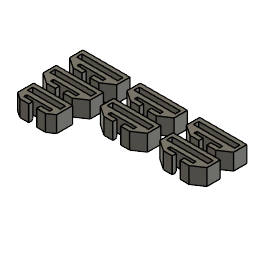
syringe pump (Autodesk Fusion 360 archive; units mm, degrees)
design "stringe pump 2"
Autodesk Fusion 360 part; units mm, degrees
sketch "Sketch1" plane through (0, 0, 0) normal (0, 1, 0) x (1, 0, 0)
  line L0 (0, 0) -> (19, 0)
  line L1 (19, -2.5) -> (0, -2.5)
  line L2 (0, 0) -> (19, 0)
  line L3 (-2, -4.5) -> (-2, 2)
  line L4 (-2, 2) -> (21, 2)
  line L5 (21, 2) -> (21, -4.5)
  line L6 (21, -4.5) -> (15.75, -8)
  line L7 (-2, -4.5) -> (3.25, -8)
  line L8 (15.75, -6) -> (15.75, -4.65)
  line L9 (3.25, -4.65) -> (3.25, -6)
  line L10 (3.25, -6) -> (7.5, -6)
  line L11 (15.75, -6) -> (11.5, -6)
  line L12 (3.25, -8) -> (7.5, -8)
  line L13 (11.5, -8) -> (15.75, -8)
  line L14 (3.25, -8) -> (7.5, -8)
  line L15 (11.5, -8) -> (15.75, -8)
  line L16 (15.75, -6) -> (11.5, -6)
  line L17 (7.5, -6) -> (3.25, -6)
  line L18 (3.25, -6) -> (7.5, -6)
  line L19 (11.5, -6) -> (15.75, -6)
  line L20 (7.5, -8) -> (11.5, -8)
  line L21 (15.75, -6) -> (15.75, -4.65)
  line L22 (15.75, -4.65) -> (3.25, -4.65)
  line L23 (3.25, -4.65) -> (3.25, -6)
  line L24 (0, 0) -> (-0.5, 0)
  line L25 (-0.5, 0) -> (-0.5, -2.5)
  line L26 (-0.5, -2.5) -> (-0.2, -2.5)
  line L27 (19, 0) -> (19.5, 0)
  line L28 (19.5, 0) -> (19.5, -2.5)
  line L29 (19.5, -2.5) -> (19, -2.5)
  line L30 (7.5, -6) -> (7.6, -6)
  line L31 (7.6, -6) -> (7.6, -8)
  line L32 (7.6, -8) -> (7.5, -8)
  line L33 (11.5, -6) -> (11.4, -6)
  line L34 (11.4, -6) -> (11.4, -8)
  line L35 (11.4, -8) -> (11.5, -8)
  line L36 (3.25, -6) -> (7.6, -6)
  line L37 (11.4, -6) -> (15.75, -6)
  line L38 (0, -2.5) -> (-0.2, -2.5)
  dimension "d28" = 1.35
  dimension "d29" = 0.5
  dimension "d30" = 0.5
  dimension "d31" = 0.1
  dimension "d32" = 0.1
  constraint horizontal L0
  constraint coincident L0.start L2.start
  constraint horizontal L2
  constraint vertical L3
  constraint horizontal L4
  constraint vertical L5
  constraint horizontal L12
  constraint horizontal L16
  constraint horizontal L18
  constraint vertical L8
  constraint vertical L9
  constraint collinear L16 L17
  constraint collinear L18 L19
  constraint horizontal L36
  constraint vertical L21
  constraint horizontal L22
  constraint vertical L23
  constraint horizontal L24
  constraint vertical L25
  constraint horizontal L26
  constraint horizontal L27
  constraint vertical L28
  constraint horizontal L29
  constraint horizontal L30
  constraint vertical L31
  constraint horizontal L32
  constraint horizontal L33
  constraint vertical L34
  constraint horizontal L35
  constraint collinear L36 L37
  constraint parallel L26 L38
  measures "d28" distance of L9.end L9.start
  measures "d29" distance of L0.start L24.end
  measures "d30" distance of L0.end L27.end
  measures "d31" distance of L10.end L30.end
  measures "d32" distance of L11.end L33.end
extrude "Extrude1" add sketch "Sketch1" along normal blind 8 contours L3 L4 L5 L6 L7 L8 L9 L10 L11 L12 L13 L14 L15 L16 L17 L18 L19 L20 L21 L22 L23 L30 L31 L32 L33 L34 L35 L36 L37 makes body 1
fillet "Fillet1" radius 2.5 1 edges at (9.5, 0, 0) on bodies 1
fillet "Fillet3" radius 1 2 edges at (9.5, 0, 2.5) (9.5, 0, 4.65) on bodies 1
fillet "Fillet2" radius 1 4 edges at (13.575, 0, 6) (5.425, 0, 6) (15.75, 0, 4.825) (3.25, 0, 4.825) on bodies 1
move_body "Move2" bodies 1 to x (1, 0, 0) y (0, 1, 0) z (0, 0, 1) at (0, 0, -17)
move_body "Move3" bodies 1 to x (1, 0, 0) y (0, 1, 0) z (0, 0, 1) at (-10, 0, 0)
copy_body "CopyPasteBodies1" bodies 1 makes body 2
move_body "Move4" bodies 2 to x (1, 0, 0) y (0, 1, 0) z (0, 0, 1) at (28, 0, 0)
copy_body "CopyPasteBodies2" bodies 2 makes body 3
move_body "Move5" bodies 3 to x (1, 0, 0) y (0, 1, 0) z (0, 0, 1) at (29, 0, 0)
copy_body "CopyPasteBodies3" bodies 1 2 3 makes body 4 makes body 5 makes body 6
move_body "Move6" bodies 4 5 6 to x (1, 0, 0) y (0, 1, 0) z (0, 0, 1) at (0, 0, 13)
copy_body "CopyPasteBodies4" bodies 1 makes body 7
move_body "Move7" bodies 7 to x (1, 0, 0) y (0, 1, 0) z (0, 0, 1) at (0, 0, 26)
sketch "Sketch2" plane through (0, 8, 0) normal (0, 1, 0) x (-1, 0, 0)
  line L0 (10.5, 9) -> (-9.5, 9)
  line L1 (-9.5, 9) -> (-9.5, 11.5)
  line L2 (-9.5, 11.5) -> (10.5, 11.5)
  line L3 (10.5, 11.5) -> (10.5, 9)
  line L4 (-1.4, 17) -> (-1.5, 17)
  line L5 (-1.5, 17) -> (-5.75, 17)
  line L6 (-5.75, 17) -> (-11, 13.5)
  line L7 (-11, 13.5) -> (-11, 7)
  line L8 (-11, 7) -> (12, 7)
  line L9 (12, 7) -> (12, 13.5)
  line L10 (12, 13.5) -> (6.75, 17)
  line L11 (6.75, 17) -> (2.5, 17)
  line L12 (2.5, 17) -> (2.4, 17)
  line L13 (2.4, 17) -> (2.4, 15)
  line L14 (2.4, 15) -> (6.75, 15)
  line L15 (6.75, 15) -> (6.75, 13.65)
  line L16 (6.75, 13.65) -> (-5.75, 13.65)
  line L17 (-5.75, 13.65) -> (-5.75, 15)
  line L18 (-5.75, 15) -> (-1.4, 15)
  line L19 (-1.4, 15) -> (-1.4, 17)
  line L20 (10.5, 7) -> (-9.5, 7)
  line L21 (-9.5, 7) -> (-9.5, 14.5)
  line L22 (-9.5, 14.5) -> (10.5, 14.5)
  line L23 (10.5, 14.5) -> (10.5, 7)
  line L24 (10.5, 7) -> (10, 7)
  line L25 (10, 7) -> (10, 14.5)
  line L26 (10, 14.5) -> (10.5, 14.5)
  line L27 (10.5, 14.5) -> (10.5, 7)
  line L28 (-9.5, 7) -> (-9, 7)
  line L29 (-9, 7) -> (-9, 14.5)
  line L30 (-9, 14.5) -> (-9.5, 14.5)
  line L31 (-9.5, 14.5) -> (-9.5, 7)
  line L32 (-9, 7) -> (-7.5, 7)
  line L33 (-7.5, 7) -> (-7.5, 12.5)
  line L34 (-7.5, 12.5) -> (-9, 12.5)
  line L35 (-9, 12.5) -> (-9, 7)
  line L36 (10, 7) -> (8.5, 7)
  line L37 (8.5, 7) -> (8.5, 12.5)
  line L38 (8.5, 12.5) -> (10, 12.5)
  line L39 (10, 12.5) -> (10, 7)
  line L40 (-9.5, 14.5) -> (-9, 14.5)
  line L41 (-9, 14.5) -> (-9, 15.5)
  line L42 (-9, 15.5) -> (-9.5, 15.5)
  line L43 (-9.5, 15.5) -> (-9.5, 14.5)
  line L44 (10.5, 14.5) -> (10, 14.5)
  line L45 (10, 14.5) -> (10, 15.5)
  line L46 (10, 15.5) -> (10.5, 15.5)
  line L47 (10.5, 15.5) -> (10.5, 14.5)
  dimension "d35" = 0.5
  dimension "d36" = 0.5
  dimension "d39" = 1.5
  dimension "d40" = 1.5
  dimension "d41" = 1
  constraint horizontal L20
  constraint vertical L21
  constraint horizontal L22
  constraint vertical L23
  constraint coincident L6 L21.end
  constraint coincident L8 L20.start
  constraint horizontal L24
  constraint vertical L25
  constraint horizontal L26
  constraint vertical L27
  constraint horizontal L28
  constraint vertical L29
  constraint horizontal L30
  constraint vertical L31
  constraint horizontal L32
  constraint vertical L33
  constraint horizontal L34
  constraint vertical L35
  constraint horizontal L36
  constraint vertical L37
  constraint horizontal L38
  constraint vertical L39
  constraint horizontal L40
  constraint vertical L41
  constraint horizontal L42
  constraint vertical L43
  constraint horizontal L44
  constraint vertical L45
  constraint horizontal L46
  constraint vertical L47
  measures "d35" distance of L20.start L24.end
  measures "d36" distance of L20.end L28.end
  measures "d39" distance of L28.end L32.end
  measures "d40" distance of L24.end L36.end
  measures "d41" distance of L22.end L46.end
extrude "Extrude3" cut sketch "Sketch2" against normal blind 8 contours L0 L8 L20 L23 L24 L25 L27 L39 | L0 L2 L3 L23 L25 L27 L39 | L3 L8 L9 L10 L23 L27 | L2 L22 L23 L25 L26 L27 L39 L44 | L10 L22 L26 L44 L45 | L10 L45 L46 L47 | L0 L8 L20 L21 L28 L29 L31 L35 | L0 L1 L2 L21 L29 L31 L35 | L1 L6 L7 L8 L21 L31 | L2 L21 L22 L29 L30 L31 L35 L40 | L6 L22 L30 L40 L41 | L6 L41 L42 L43 bodies 7 makes body 8 at (-3.6667, 2.6667, 7)
extrude "Extrude4" add sketch "Sketch2" against normal blind 8 contours L0 L8 L20 L25 L36 L37 L39 | L0 L2 L25 L37 L39 | L2 L25 L37 L38 L39 | L0 L8 L20 L29 L32 L33 L35 | L0 L2 L29 L33 L35 | L2 L29 L33 L34 L35 bodies 7 8
